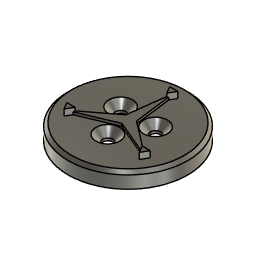
holder_round_25mm (Autodesk Fusion 360 design; units mm, degrees)
Autodesk Fusion 360 part; units mm, degrees
sketch "Sketch1" plane through (0, 0, 0) normal (0, 0, 1) x (1, 0, 0) in component "Round Holder  parametric"
  circle A0 centre (0, 0) radius 19.25
  line L0 (0, 11.547) -> (-10, 5.7735)
  line L1 (-10, 5.7735) -> (-10, -5.7735)
  line L2 (-10, -5.7735) -> (0, -11.547)
  line L3 (0, -11.547) -> (10, -5.7735)
  line L4 (10, -5.7735) -> (10, 5.7735)
  line L5 (10, 5.7735) -> (0, 11.547)
  line L6 (-10.3, 5.9467) -> (-10.3, -5.9467)
  line L7 (-10.3, -5.9467) -> (0, -11.8934)
  line L8 (0, -11.8934) -> (10.3, -5.9467)
  line L9 (10.3, -5.9467) -> (10.3, 5.9467)
  line L10 (10.3, 5.9467) -> (0, 11.8934)
  line L11 (0, 11.8934) -> (-10.3, 5.9467)
  circle A1 centre (0, 0) radius 14 construction
  line L12 (0, 12.5) -> (1.299, 14.75)
  line L13 (1.299, 14.75) -> (-1.299, 14.75)
  line L14 (-1.299, 14.75) -> (0, 12.5)
  line L15 (-1.7321, 1) -> (0, -2) construction
  line L16 (0, -2) -> (1.7321, 1) construction
  line L17 (1.7321, 1) -> (-1.7321, 1) construction
  line L18 (-1.7321, 1) -> (0, 14.75)
  line L19 (0, 14.75) -> (1.7321, 1)
  line L20 (0, -2) -> (-12.7739, -7.375)
  line L21 (-12.7739, -7.375) -> (-1.7321, 1)
  line L22 (1.7321, 1) -> (12.7739, -7.375)
  line L23 (12.7739, -7.375) -> (0, -2)
  line L24 (-10.8253, -6.25) -> (-13.4234, -6.25)
  line L25 (-13.4234, -6.25) -> (-12.1244, -8.5)
  line L26 (-12.1244, -8.5) -> (-10.8253, -6.25)
  line L27 (10.8253, -6.25) -> (12.1244, -8.5)
  line L28 (12.1244, -8.5) -> (13.4234, -6.25)
  line L29 (13.4234, -6.25) -> (10.8253, -6.25)
  line L30 (0, 0) -> (0, 14.75) construction
  circle A2 centre (0, 0) radius 6.5 construction
  circle A3 centre (0, 0) radius 6.5 construction
  circle A4 centre (0, -6.5) radius 1.65
  circle A5 centre (5.6292, 3.25) radius 1.65
  circle A6 centre (-5.6292, 3.25) radius 1.65
  line L31 (0, -11.8934) -> (0, -2) construction
  circle A7 centre (0, 0) radius 12.5 construction
  point P0 (0, 14)
  dimension "d46" = 38.5
  dimension "d54" = 10
  dimension "d55" = 0.3
  dimension "d72" = 1.5
  dimension "d73" = 1
  dimension "d82" = 360
  dimension "d84" = 360
  dimension "d86" = 13
  dimension "d90" = 13
  dimension "d91" = 3.3
  dimension "d93" = 360
  dimension "d109" = 25
  constraint coincident A0.centre A1.centre
  constraint concentric A0 A1
  constraint coincident A1 P0
  constraint parallel L13 L17
  constraint midpoint L13 L18.end
  constraint coincident L19 L16.end
  constraint coincident L20 L15.end
  constraint coincident L15.end L20
  constraint equal L22 L23
  constraint coincident L16.end L17.start
  constraint horizontal L13
  constraint coincident L12.start L30
  constraint coincident A2 A4.centre
  constraint vertical L9
  constraint coincident A4.centre L31
  constraint concentric A1 A7
  constraint coincident L12.start A7
  measures "d46" diameter of A0
  measures "d54" distance of A0.centre L5
  measures "d72" distance of L12.start P0
  measures "d73" distance of A0.centre L17
  measures "d86" diameter of A2
  measures "d90" diameter of A3
  measures "d91" diameter of A4
  measures "d109" diameter of A7
extrude "Extrude1" add sketch "Sketch1" along normal blind 5 contours A0 | L0 L1 L2 L3 L4 L5 L18 L19 L20 L21 L22 L23 | L0 L5 L10 L11 L18 L19 | L0 L1 L18 L21 | L0 L1 L6 L11 L18 L21 | L4 L5 L9 L10 L19 L22 | L4 L5 L19 L22 | L10 L11 L12 L14 L18 L19 | L1 L2 L6 L7 L20 L21 | L12 L14 L18 L19 | L13 L14 L18 | L3 L4 L8 L9 L22 L23 | L12 L13 L19 | L6 L7 L20 L21 L24 L26 | L8 L9 L22 L23 L27 L29 | L2 L3 L20 L23 | L2 L3 L7 L8 L20 L23 | L20 L21 L24 L26 | L21 L24 L25 | L22 L28 L29 | L22 L23 L27 L29 | L20 L25 L26 | L23 L27 L28 | A4 | A5 | A6 in component "Round Holder  parametric"
extrude "Extrude10" cut sketch "Sketch1" along normal blind 2 contours L0 L1 L2 L3 L4 L5 L18 L19 L20 L21 L22 L23 | L0 L5 L10 L11 L18 L19 | L0 L1 L18 L21 | L0 L1 L6 L11 L18 L21 | L4 L5 L9 L10 L19 L22 | L4 L5 L19 L22 | L1 L2 L6 L7 L20 L21 | L3 L4 L8 L9 L22 L23 | L2 L3 L20 L23 | L2 L3 L7 L8 L20 L23 | A4 | A5 | A6 in component "Round Holder  parametric"
extrude "Extrude11" add sketch "Sketch1" along normal blind 0.8 from surface at 5 contours L0 L1 L2 L3 L4 L5 L18 L19 L20 L21 L22 L23 | L0 L5 L10 L11 L18 L19 | L10 L11 L12 L14 L18 L19 | L1 L2 L6 L7 L20 L21 | L12 L14 L18 L19 | L3 L4 L8 L9 L22 L23 | L6 L7 L20 L21 L24 L26 | L8 L9 L22 L23 L27 L29 | L20 L21 L24 L26 | L22 L23 L27 L29 in component "Round Holder  parametric"
extrude "Extrude12" add sketch "Sketch1" along normal blind 2 from surface at 5 contours L12 L14 L18 L19 | L13 L14 L18 | L12 L13 L19 | L20 L21 L24 L26 | L21 L24 L25 | L22 L28 L29 | L22 L23 L27 L29 | L20 L25 L26 | L23 L27 L28 in component "Round Holder  parametric"
extrude "Extrude13" cut sketch "Sketch1" along normal through all contours A4 | A5 | A6 in component "Round Holder  parametric"
chamfer "Chamfer3" distance 2.2 angle 45 3 edges at (-1.5383, -5.9033, 5) (-7.1675, 3.8467, 5) (4.0908, 3.8467, 5) in component "Round Holder  parametric"
chamfer "Chamfer4" distance 1 angle 45 1 edges at (-17.9473, -6.9611, 5) in component "Round Holder  parametric"
component "Round Holder  parametric" placed x (1, 0, 0) y (0, 1, 0) z (0, 0, 1) at (0, 0, 0)
equation "d46 = slide_diam + 13 mm"
equation "slide_diam = 25.5 mm"
equation "print_compensation = 0.5 mm"
equation "d109 = slide_diam - print_compensation"
